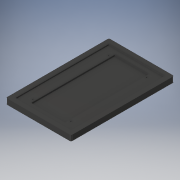
# Autodesk Inventor part: Cover
Saved by Autodesk Inventor 2019.4 (Build 234330000, 330)
## iProperties
Created: 2021-01-28
Part Number: Cover
Material: Acetal Resin, Black
Document SubType Name: Modeling
Designer: caleb
Density: 1.425 g/cm^3
Appearance: Smooth - Black
Author: caleb
Autodesk Inventor part; units mm, degrees
ref_plane "YZ Plane" through (0, 0, 0) normal (1, 0, 0) x (0, 1, 0)
ref_plane "XZ Plane" through (0, 0, 0) normal (0, 1, 0) x (-1, 0, 0)
ref_plane "XY Plane" through (0, 0, 0) normal (0, 0, 1) x (1, 0, 0)
sketch "Sketch1" plane through (0, 0, 0) normal (0, 1, 0) x (-1, 0, 0)
  line L0 (-76.2, 120.65) -> (76.2, 120.65)
  line L1 (76.2, 120.65) -> (76.2, -120.65)
  line L2 (76.2, -120.65) -> (-76.2, -120.65)
  line L3 (-76.2, -120.65) -> (-76.2, 120.65)
  line L4 (-76.2, 120.65) -> (76.2, -120.65) construction
  line L5 (76.2, 120.65) -> (-76.2, -120.65) construction
  point P0 (0, 0)
  dimension "d0" = 241.3
  dimension "d1" = 152.4
  constraints: 12 end point, 2 midpoint, 2 parallel, 1 horizontal, 1 perpendicular
  measures "d0" distance of L0.end L1.end
  measures "d1" distance of L1.end L2.end
extrude "Extrusion1" add sketch "Sketch1" along normal blind 12.7
sketch "Sketch2" plane through (0, 12.7, 0) normal (0, 1, 0) x (1, 0, 0)
  line L0 (65.0875, -109.5375) -> (-65.0875, -109.5375)
  line L1 (-65.0875, -109.5375) -> (-65.0875, 109.5375)
  line L2 (-65.0875, 109.5375) -> (65.0875, 109.5375)
  line L3 (65.0875, 109.5375) -> (65.0875, -109.5375)
  line L4 (65.0875, -109.5375) -> (-65.0875, 109.5375) construction
  line L5 (-65.0875, -109.5375) -> (65.0875, 109.5375) construction
  point P0 (0, 0)
  dimension "d4" = 219.075
  dimension "d5" = 130.175
  constraints: 12 end point, 2 midpoint, 2 parallel, 1 horizontal, 1 perpendicular
  measures "d4" distance of L0.end L1.end
  measures "d5" distance of L1.end L2.end
extrude "Extrusion2" cut sketch "Sketch2" against normal blind 3.175
sketch "Sketch3" plane through (0, 9.525, 0) normal (0, 1, 0) x (1, 0, 0)
  line L0 (39.6875, -98.1075) -> (-39.6875, -98.1075)
  line L1 (-39.6875, -98.1075) -> (-39.6875, 98.1075)
  line L2 (-39.6875, 98.1075) -> (39.6875, 98.1075)
  line L3 (39.6875, 98.1075) -> (39.6875, -98.1075)
  line L4 (39.6875, -98.1075) -> (-39.6875, 98.1075) construction
  line L5 (-39.6875, -98.1075) -> (39.6875, 98.1075) construction
  line L6 (65.0875, -109.5375) -> (-65.0875, -109.5375) projected
  line L7 (-65.0875, 109.5375) -> (65.0875, 109.5375) projected
  line L8 (-65.0875, -109.5375) -> (-65.0875, 109.5375) projected
  point P0 (0, 0)
  dimension "d8" = 11.43
  dimension "d9" = 25.4
  constraints: 12 end point, 2 midpoint, 2 parallel, 1 horizontal, 1 perpendicular
  measures "d8" distance between parallel lines of L6 L0
  measures "d9" distance between parallel lines of L8 L1
extrude "Extrusion3" cut sketch "Sketch3" against normal blind 3.81
sketch "Sketch4" plane through (0, 9.525, 0) normal (0, 1, 0) x (1, 0, 0)
  line L0 (-65.0875, -109.5375) -> (-65.0875, 109.5375) projected
  line L1 (65.0875, -109.5375) -> (-65.0875, -109.5375) projected
  point P0 (0, 0)
  point P1 (-44.45, -88.9)
  point P2 (-44.45, 88.9)
  point P3 (44.45, -88.9)
  point P4 (44.45, 88.9)
  dimension "d12" = 20.6375
  dimension "d13" = 20.6375
  dimension "d16" = 177.8
  dimension "d19" = 88.9
  constraints: 1 horizontal, 1 vertical, 3 other
  measures "d12" distance from line of L0 point (-44.45, -88.9)
  measures "d13" distance from line of L1 point (-44.45, -88.9)
  measures "d16" distance of point (-44.45, -88.9) point (-44.45, 88.9)
  measures "d19" distance of point (-44.45, -88.9) point (44.45, -88.9)
hole "Hole1" at (-44.45, 9.525, 88.9) at (-44.45, 9.525, -88.9) at (44.45, 9.525, 88.9) at (44.45, 9.525, -88.9) direction (0, -1, 0) diameter 3.4036 end through all clearance for "Flat Head Machine Screw" size "M3" standard "Ansi Metric M Profile"
fillet "Fillet1" radius 3.175 4 edges at (-76.2, 6.35, 120.65) (76.2, 6.35, 120.65) (-76.2, 6.35, -120.65) (76.2, 6.35, -120.65)
body "Solid1"
